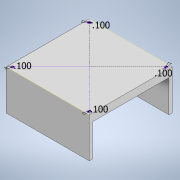
# Autodesk Inventor part: TurntableBase2
Saved by Autodesk Inventor 2020 (Build 240168000, 168)
## iProperties
Created: 2022-02-25
Part Number: TurntableBase2
Material: Generic
Document SubType Name: Modeling
Designer: danie
Density: 1 g/cm^3
Appearance: Default
Author: danie
Autodesk Inventor part; units mm, degrees
ref_plane "YZ Plane" through (0, 0, 0) normal (1, 0, 0) x (0, 1, 0)
ref_plane "XZ Plane" through (0, 0, 0) normal (0, 1, 0) x (-1, 0, 0)
ref_plane "XY Plane" through (0, 0, 0) normal (0, 0, 1) x (1, 0, 0)
sketch "Sketch1" plane through (0, 0, 0) normal (0, 1, 0) x (-1, 0, 0)
  line L0 (0, 0) -> (-82.55, 0)
  line L1 (-82.55, 0) -> (-82.55, -82.55)
  line L2 (-82.55, -82.55) -> (0, -82.55)
  line L3 (0, -82.55) -> (0, 0)
  dimension "d0" = 82.55
  dimension "d1" = 82.55
  constraints: 8 end point, 2 parallel, 1 horizontal, 1 perpendicular
  measures "d0" distance of L2.end L1.end
  measures "d1" distance of L1.end L0.end
extrude "Extrusion1" add sketch "Sketch1" along normal blind 7.62
sketch "Sketch2" plane through (0, 0, 0) normal (0, -1, 0) x (1, 0, 0)
  line L0 (82.55, 0) -> (82.55, -82.55) projected
  line L1 (82.55, 0) -> (0, 0)
  line L2 (0, 0) -> (0, -3.175)
  line L3 (0, -3.175) -> (82.55, -3.175)
  line L4 (82.55, -3.175) -> (82.55, 0)
  line L5 (82.55, -82.55) -> (0, -82.55)
  line L6 (0, -82.55) -> (0, -79.375)
  line L7 (0, -79.375) -> (82.55, -79.375)
  line L8 (82.55, -79.375) -> (82.55, -82.55)
  dimension "d4" = 82.55
  dimension "d5" = 3.175
  dimension "d6" = 82.55
  dimension "d7" = 3.175
  constraints: 16 end point, 4 parallel, 2 horizontal, 2 perpendicular
  measures "d4" distance of L3.end L2.end
  measures "d5" distance of L2.end L1.end
  measures "d6" distance of L6.end L7.end
  measures "d7" distance of L5.end L6.end
extrude "Extrusion2" add sketch "Sketch2" along normal blind 32.0802
sketch "Sketch3" plane through (0, 7.62, 0) normal (0, 1, 0) x (1, 0, 0)
  line L0 (0, 82.55) -> (82.55, 82.55) construction
  line L1 (0, 0) -> (82.55, 82.55) construction
  line L2 (82.55, 0) -> (0, 0) construction
  line L3 (0, 82.55) -> (82.55, 0) construction
  circle A0 centre (3.0661, 3.0077) radius 1.27
  circle A1 centre (3.0661, 79.5423) radius 1.27
  circle A2 centre (79.4839, 79.5423) radius 1.27
  circle A3 centre (79.4839, 3.0077) radius 1.27
  line L4 (3.0661, 3.0077) -> (79.4839, 79.5423) construction
  line L5 (3.0661, 79.5423) -> (79.4839, 3.0077) construction
  dimension "d14" = 2.54
  dimension "d15" = 2.54
  dimension "d16" = 2.54
  dimension "d17" = 2.54
  constraints: 8 end point, 4 centre point
  measures "d14" diameter of A0
  measures "d15" diameter of A1
  measures "d16" diameter of A2
  measures "d17" diameter of A3
body "Solid1"
